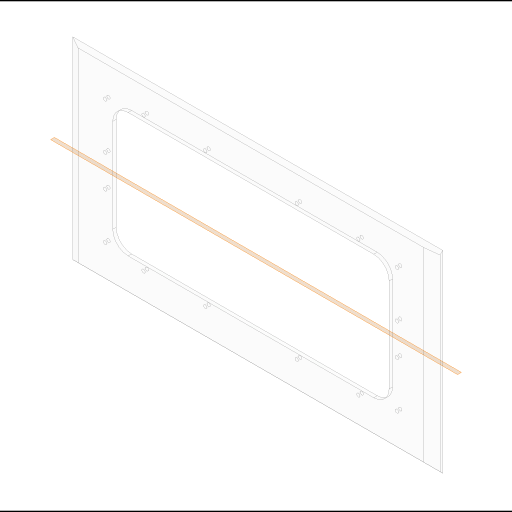
# Autodesk Inventor part: Wind Tunnel Test Section Front
Saved by Autodesk Inventor 2023 (Build 270158000, 158)
## iProperties
Created: 2022-03-05
Part Number: Wind Tunnel Test Section Front
Material: Polycarbonate, Clear
Document SubType Name: Modeling
Designer: kamer
Density: 1.2 g/cm^3
Appearance: Polycarbonate - Clear
Author: kamer
Autodesk Inventor part; units mm, degrees
ref_plane "YZ Plane" through (0, 0, 0) normal (1, 0, 0) x (0, 1, 0)
ref_plane "XY Plane" through (0, 0, 0) normal (0, 0, 1) x (1, 0, 0)
sketch "Sketch1" plane through (0, 0, 0) normal (0, 0, 1) x (1, 0, 0)
  line L0 (0, 0) -> (609.6, 0)
  line L1 (609.6, 0) -> (609.6, 317.881)
  line L2 (609.6, 317.881) -> (0, 317.881)
  line L3 (0, 317.881) -> (0, 0)
  dimension "d0" = 609.6
  dimension "d1" = 317.881
  constraints: 8 end point, 2 parallel, 1 horizontal, 1 perpendicular
  measures "d0" distance of L1.end L2.end
  measures "d1" distance of L0.end L1.end
extrude "Extrusion1" add sketch "Sketch1" along normal blind 5.7658
sketch "Sketch2" plane through (0, 317.881, 0) normal (0, 1, 0) x (1, 0, 0)
  line L0 (609.6, 0) -> (0, 0) projected
  line L1 (0, 0) -> (0, -5.7658) projected
  line L2 (609.6, -5.7658) -> (0, -5.7658) projected
  line L3 (609.6, 0) -> (609.6, -5.7658) projected
  line L4 (0, 0) -> (609.6, 0) projected
  line L5 (0, 0) -> (14.4594, -5.7658)
  line L6 (0, -5.7658) -> (609.6, -5.7658) projected
  line L7 (14.4594, -5.7658) -> (14.4594, 0)
  line L8 (14.4594, -5.7658) -> (20.2252, -5.7658) construction
  dimension "d4" = 21.74
  dimension "d5" = 90
  constraints: 6 end point, 2 point on line, 1 horizontal, 1 perpendicular
  measures "d4" angle of L5 L0
  measures "d5" angle of L8 L7
extrude "Extrusion2" cut sketch "Sketch2" against normal through all contours L5 L2 L1
sketch "Sketch3" plane through (609.6, 0, 0) normal (1, 0, 0) x (0, 0, -1)
  line L0 (0, 0) -> (0, 317.881) projected
  line L1 (0, 317.881) -> (-5.7658, 317.881) projected
  line L2 (-5.7658, 0) -> (-5.7658, 317.881) projected
  line L3 (0, 0) -> (-5.7658, 0) projected
  line L4 (0, 0) -> (-5.7658, 0) projected
  line L5 (0, 0) -> (-5.7658, 5.7658)
  line L6 (-5.7658, 0) -> (-5.7658, 317.881) projected
  line L7 (0, 0) -> (8.1541, 0) construction
  line L8 (0, 317.881) -> (-5.7658, 317.881) projected
  line L9 (0, 317.881) -> (-5.7658, 312.1152)
  line L10 (0, 317.881) -> (8.1541, 317.881) construction
  dimension "d8" = 135
  dimension "d9" = 135
  constraints: 8 end point, 2 equal length, 2 horizontal, 2 point on line
  measures "d8" angle of L7 L5
  measures "d9" angle of L9 L10
extrude "Extrusion3" cut sketch "Sketch3" against normal through all contours L3 L2 L5 | L9 L2 L1
ref_plane "Center Plane" through (0, 158.9405, 0) normal (0, 1, 0) x (-1, 0, 0)
sketch "Sketch4" plane through (0, 158.9405, 0) normal (0, 1, 0) x (-1, 0, 0)
  line L0 (-14.4594, 5.7658) -> (0, 0) projected
  line L1 (-609.6, 5.7658) -> (-14.4594, 5.7658) projected
  line L2 (-609.6, 0) -> (-609.6, 5.7658) projected
  line L3 (-609.6, 0) -> (0, 0) projected
  line L4 (-609.6, 5.7658) -> (-584.2, 5.7658) construction
  line L5 (-609.6, 5.7658) -> (-14.4594, 5.7658) construction
  line L6 (-584.2, 5.7658) -> (-609.6, 4.4413)
  point P0 (0, 0)
  dimension "d13" = 25.4
  dimension "d14" = 2.985
  constraints: 4 end point, 2 point on line
  measures "d13" distance of L1.start L4.end
  measures "d14" angle of L4 L6
extrude "Extrusion4" cut sketch "Sketch4" against normal through all both and the other way through all contours L6 L2 L1
sketch "Sketch5" plane through (0, 0, 5.7658) normal (0, 0, 1) x (1, 0, 0)
  line L0 (97.0094, 261.3152) -> (501.65, 261.3152)
  line L1 (527.05, 235.9152) -> (527.05, 81.9658)
  line L2 (501.65, 56.5658) -> (97.0094, 56.5658)
  line L3 (71.6094, 81.9658) -> (71.6094, 235.9152)
  line L4 (584.2, 312.1152) -> (14.4594, 312.1152) projected
  line L5 (14.4594, 5.7658) -> (584.2, 5.7658) projected
  line L6 (584.2, 5.7658) -> (584.2, 312.1152) projected
  line L7 (14.4594, 312.1152) -> (14.4594, 5.7658) projected
  arc A0 (97.0094, 261.3152) -> (71.6094, 235.9152) centre (97.0094, 235.9152) ccw
  arc A1 (527.05, 235.9152) -> (501.65, 261.3152) centre (501.65, 235.9152) ccw
  arc A2 (501.65, 56.5658) -> (527.05, 81.9658) centre (501.65, 81.9658) ccw
  arc A3 (71.6094, 81.9658) -> (97.0094, 56.5658) centre (97.0094, 81.9658) ccw
  point P0 (0, 0)
  dimension "d18" = 50.8
  dimension "d19" = 50.8
  dimension "d20" = 57.15
  dimension "d21" = 57.15
  dimension "d22" = 25.4
  constraints: 8 end point, 8 point on circle, 8 tangent, 4 centre point, 3 equal radius, 2 parallel, 1 horizontal, 1 perpendicular
  measures "d18" distance between parallel lines of L0 L4
  measures "d19" distance between parallel lines of L5 L2
  measures "d20" distance between parallel lines of L6 L1
  measures "d21" distance between parallel lines of L7 L3
  measures "d22" radius of A0
extrude "Extrusion5" cut sketch "Sketch5" against normal through all contours L0 A1 L1 A2 L2 A3 L3 A0
sketch "Sketch6" plane through (0, 0, 5.7658) normal (0, 0, 1) x (1, 0, 0)
  circle A0 centre (539.75, 56.5658) radius 2.7559
  circle A1 centre (539.75, 132.7658) radius 2.7559
  circle A2 centre (539.75, 185.1152) radius 2.75
  circle A3 centre (539.75, 261.3152) radius 2.7559
  line L0 (527.05, 235.9152) -> (527.05, 81.9658) projected
  line L1 (501.65, 56.5658) -> (97.0094, 56.5658) projected
  circle A4 centre (58.9026, 56.5658) radius 2.7559
  circle A5 centre (58.9026, 132.7658) radius 2.7559
  circle A6 centre (58.9026, 185.1152) radius 2.75
  circle A7 centre (58.9026, 261.3152) radius 2.7559
  circle A8 centre (476.25, 47.6758) radius 2.7559
  circle A9 centre (374.65, 47.6758) radius 2.7559
  circle A10 centre (224.0026, 47.6758) radius 2.7559
  circle A11 centre (122.4026, 47.6758) radius 2.7559
  circle A12 centre (476.25, 270.2052) radius 2.7559
  circle A13 centre (374.65, 270.2052) radius 2.7559
  circle A14 centre (224.0026, 270.2052) radius 2.7559
  circle A15 centre (122.4026, 270.2052) radius 2.7559
  point P0 (0, 0)
  dimension "d25" = 5.5118
  dimension "d26" = 5.5118
  dimension "d27" = 5.5
  dimension "d28" = 5.5118
  dimension "d29" = 12.7
  dimension "d30" = 25.4
  dimension "d31" = 76.2
  dimension "d32" = 52.3494
  dimension "d33" = 76.2
  dimension "d34" = 12.7
  dimension "d35" = 12.7
  dimension "d36" = 12.7
  dimension "d39" = 480.8474
  dimension "d44" = 5.5118
  dimension "d45" = 5.5118
  dimension "d46" = 5.5118
  dimension "d48" = 63.5
  dimension "d49" = 8.89
  dimension "d50" = 8.89
  dimension "d51" = 8.89
  dimension "d53" = 101.6
  dimension "d54" = 150.6474
  dimension "d55" = 5.5118
  dimension "d56" = 101.6
  dimension "d57" = 8.89
  dimension "d63" = 222.5294
  constraints: 16 centre point, 1 horizontal, 1 vertical, 16 other
  measures "d25" diameter of A0
  measures "d26" diameter of A1
  measures "d27" diameter of A2
  measures "d28" diameter of A3
  measures "d29" distance from line of L0 A0.centre
  measures "d30" vertical distance of L0.end A0.centre
  measures "d31" distance of A1.centre A0.centre
  measures "d32" distance of A2.centre A1.centre
  measures "d33" distance of A2.centre A3.centre
  measures "d34" distance from line of L0 A1.centre
  measures "d35" distance from line of L0 A2.centre
  measures "d36" distance from line of A3.centre L0
  measures "d39" distance of A0.centre A4.centre
  measures "d44" diameter of A8
  measures "d45" diameter of A9
  measures "d46" diameter of A10
  measures "d48" horizontal distance of A0.centre A8.centre
  measures "d49" distance from line of L1 A8.centre
  measures "d50" distance from line of A9.centre L1
  measures "d51" distance from line of A10.centre L1
  measures "d53" distance of A8.centre A9.centre
  measures "d54" distance of A10.centre A9.centre
  measures "d55" diameter of A11
  measures "d56" distance of A11.centre A10.centre
  measures "d57" distance from line of L1 A11.centre
  measures "d63" distance of A8.centre A12.centre
extrude "Extrusion6" cut sketch "Sketch6" against normal through all
body "Solid1"
